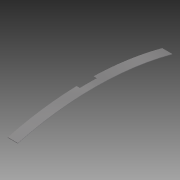
# Autodesk Inventor part: slats
Saved by Autodesk Inventor 2013 (Build 170138000, 138)
## iProperties
Created: 2012-12-18
Part Number: slats
Material: Steel, Carbon
Document SubType Name: Sheet Metal
Designer: istvan.burbank
Density: 7.87 g/cm^3
Sheet Metal Rule: Default
Flat Pattern Width: 116.84 cm
Flat Pattern Length: 7.9375 cm
Flat Pattern Area: 927.418 cm^2
Sheet Metal Width: 46.000 in
Sheet Metal Length: 3.125 in
Sheet Metal Area: 143.750 in^2
Author: istvan.burbank
Autodesk Inventor part; units mm, degrees
ref_plane "YZ Plane" through (0, 0, 0) normal (1, 0, 0) x (0, 1, 0)
sketch "Sketch7" plane through (0, 0, 0) normal (1, 0, 0) x (0, 1, 0)
  arc A0 (0, 0) -> (0, 1168.4) centre (-2201.3333, 584.2) ccw
  arc A1 (-3.175, 0) -> (-3.175, 1168.4) centre (-2201.3333, 584.2) ccw
  line L0 (-3.175, 1168.4) -> (0, 1168.4)
  line L1 (-3.175, 0) -> (0, 0)
  point P0 (76.2, 584.2)
  dimension "d36" = 1168.4
  dimension "d37" = 3.175
  dimension "d46" = 76.2
  dimension "d47" = 584.2
  dimension "d48" = 584.2
  constraints: 5 point on circle, 4 end point, 2 centre point, 1 horizontal, 1 parallel, 1 vertical alignment
  measures "d36" distance of L1.end L0.end
  measures "d37" distance of L1.start L1.end
  measures "d46" horizontal distance of L0.end point (76.2, 584.2)
  measures "d47" distance from line of point (76.2, 584.2) L0
  measures "d48" distance from line of L1 point (76.2, 584.2)
extrude "Extrusion5" add sketch "Sketch7" along normal blind 76.2
ref_plane "Work Plane2" through (0, -3.175, 1168.4) normal (0, 1, 0) x (1, 0, 0)
sketch "Sketch8" plane through (0, -3.175, 1168.4) normal (0, 1, 0) x (1, 0, 0)
  line L0 (0, 0) -> (0, 1168.4) projected
  line L1 (0, 1168.4) -> (76.2, 1168.4) projected
  line L2 (76.2, 0) -> (76.2, 1168.4) projected
  line L3 (0, 0) -> (76.2, 0) projected
  line L4 (0, 647.7) -> (25.4, 647.7)
  line L5 (25.4, 647.7) -> (25.4, 520.7)
  line L6 (25.4, 520.7) -> (0, 520.7)
  line L7 (0, 520.7) -> (0, 647.7)
  dimension "d40" = 25.4
  dimension "d41" = 127
  dimension "d42" = 520.7
  dimension "d43" = 520.7
  constraints: 8 end point, 2 parallel, 1 horizontal, 1 perpendicular, 1 point on line
  measures "d40" distance of L5.end L6.end
  measures "d41" distance of L4.end L5.end
  measures "d42" distance between parallel lines of L1 L4
  measures "d43" distance between parallel lines of L3 L6
extrude "Extrusion6" cut sketch "Sketch8" along normal through all contours L0 L4 L5 L6
ref_plane "Work Plane3" through (0, 0, 1168.4) normal (0, 1, 0) x (1, 0, 0)
equation "\"d37\" = Thickness"
equation "\"d47\" = d48"
equation "\"d42\" = d43"
equation "\"BendRadius\" = Thickness"
equation "\"BendReliefWidth\" = Thickness"
equation "\"BendReliefDepth\" = 0.5 * Thickness"
equation "\"CornerReliefSize\" = 4 * Thickness"
equation "\"MinimumRemnant\" = 2 * Thickness"
equation "\"TransitionRadius\" = BendRadius"
equation "\"JacobiRadiusSize\" = BendRadius"
equation "\"GapSize\" = Thickness"
equation "\"d2\" = BendRadius"
equation "\"Thickness\" = 3.175"
body "Solid2"
